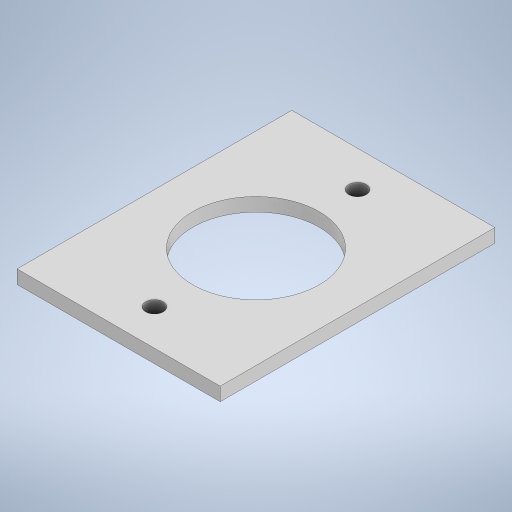
# Autodesk Inventor part: 10p_passthrough_profile
Saved by Autodesk Inventor 2023.1 (Build 271208000, 208)
## iProperties
Created: 2026-05-21
Part Number: 10p_passthrough_profile
Material: Generic
Document SubType Name: Modeling
Designer: Lars
Density: 1 g/cm^3
Appearance: Default
Author: Lars
Autodesk Inventor part; units mm, degrees
ref_plane "YZ Plane" through (0, 0, 0) normal (1, 0, 0) x (0, 1, 0)
ref_plane "XZ Plane" through (0, 0, 0) normal (0, 1, 0) x (-1, 0, 0)
ref_plane "XY Plane" through (0, 0, 0) normal (0, 0, 1) x (1, 0, 0)
sketch "Sketch1" plane through (0, 0, 0) normal (0, 1, 0) x (-1, 0, 0)
  circle A0 centre (0, 0) radius 14.05
  circle A1 centre (0, 0) radius 19.55 construction
  circle A2 centre (0, -22.55) radius 1.95
  circle A3 centre (0, 22.55) radius 1.95
  circle A4 centre (0, 22.55) radius 4.95 construction
  circle A5 centre (0, -22.55) radius 4.95 construction
  line L0 (19.55, 27.5) -> (-19.55, 27.5) construction
  line L1 (-19.55, 27.5) -> (-19.55, -27.5) construction
  line L2 (-19.55, -27.5) -> (19.55, -27.5) construction
  line L3 (19.55, -27.5) -> (19.55, 27.5) construction
  line L4 (0, 22.55) -> (0, -22.55) construction
  line L5 (-22.55, 30.5) -> (22.55, 30.5)
  line L6 (22.55, 30.5) -> (22.55, -30.5)
  line L7 (22.55, -30.5) -> (-22.55, -30.5)
  line L8 (-22.55, -30.5) -> (-22.55, 30.5)
  dimension "d0" = 28.1
  dimension "d1" = 5.5
  dimension "d2" = 3.9
  dimension "d3" = 3.9
  dimension "d4" = 22.55
  dimension "d5" = 22.55
  dimension "d6" = 3
  dimension "d7" = 3
  dimension "d8" = 3
  constraints: 18 end point, 6 centre point, 4 parallel, 4 tangent, 2 perpendicular, 1 coincident, 1 horizontal, 1 line through centre, 1 vertical, 3 other
  measures "d0" diameter of A0
  measures "d1" radial gap between concentric circles of A0 A1
  measures "d2" diameter of A2
  measures "d3" diameter of A3
  measures "d4" distance of A0.centre L4.start
  measures "d5" distance of A0.centre L4.end
  measures "d6" radial gap between concentric circles of A3 A4
  measures "d7" radial gap between concentric circles of A2 A5
  measures "d8" distance between parallel lines of L0 L5
extrude "Extrusion1" add sketch "Sketch1" along normal blind 3
equation "\"d5\" = d4"
body "Solid1"
